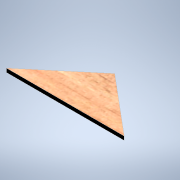
# Autodesk Inventor part: wood_front
Saved by Autodesk Inventor 2021 (Build 250183000, 183)
## iProperties
Created: 2021-08-17
Part Number: wood_front
Material: Generisch
Document SubType Name: Modeling
Designer: Tilman
Density: 1 g/cm^3
Appearance: Eloxiert - Schwarz
Author: Tilman
Autodesk Inventor part; units mm, degrees
ref_plane "YZ Plane" through (0, 0, 0) normal (1, 0, 0) x (0, 1, 0)
ref_plane "XZ Plane" through (0, 0, 0) normal (0, 1, 0) x (-1, 0, 0)
ref_plane "XY Plane" through (0, 0, 0) normal (0, 0, 1) x (1, 0, 0)
sketch "Skizze1" plane through (0, 0, 0) normal (0, 1, 0) x (-1, 0, 0)
  line L0 (0, 0) -> (-93, 0)
  line L1 (0, 0) -> (-46.5, -39)
  line L2 (-46.5, -39) -> (-93, 0)
  dimension "d0" = 93
  dimension "d4" = 39
  constraints: 6 end point, 1 equal length, 1 horizontal
  measures "d0" distance of L0.start L0.end
  measures "d4" distance from line of L0 L1.end
extrude "Extrusion1" add sketch "Skizze1" along normal blind 3
